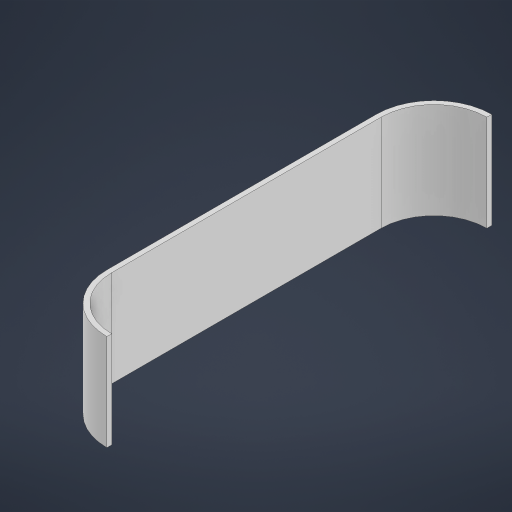
# Autodesk Inventor part: Pala
Saved by Autodesk Inventor 2023 (Build 270158000, 158)
## iProperties
Created: 2022-08-24
Part Number: Pala
Material: Generic
Document SubType Name: Modeling
Designer: river
Density: 1 g/cm^3
Appearance: Default
Author: river
Autodesk Inventor part; units mm, degrees
ref_plane "YZ Plane" through (0, 0, 0) normal (1, 0, 0) x (0, 1, 0)
ref_plane "XZ Plane" through (0, 0, 0) normal (0, 1, 0) x (-1, 0, 0)
ref_plane "XY Plane" through (0, 0, 0) normal (0, 0, 1) x (1, 0, 0)
sketch "Sketch1" plane through (0, 0, 0) normal (0, 1, 0) x (-1, 0, 0)
  line L0 (0, 0) -> (-30, 0)
  line L1 (-30, 0) -> (-30, -100)
  line L2 (-30, -100) -> (0, -100)
  line L3 (0, -100) -> (0, 0)
  line L4 (0, 0) -> (15, 0)
  line L5 (15, 0) -> (15, -55)
  line L6 (15, -55) -> (0, -55)
  line L7 (0, -55) -> (0, 0)
  circle A0 centre (7.5, 0) radius 2.5
  circle A1 centre (7.5, -20) radius 2.5
  circle A2 centre (7.5, -40) radius 2.5
  line L8 (0, -100) -> (0, -70)
  line L9 (0, -70) -> (-30, -70)
  circle A3 centre (-30, -70) radius 30
  circle A4 centre (-30, -70) radius 27.5
  line L10 (-2.5, -70) -> (-2.5, 0)
  point P0 (10, 0)
  point P1 (5, 0)
  point P2 (-30, -97.5)
  dimension "d12" = 55
  dimension "d2" = 30
  dimension "d3" = 100
  dimension "d4" = 15
  dimension "d5" = 55
  dimension "d6" = 5
  dimension "d7" = 5
  dimension "d8" = 20
  dimension "d9" = 5
  dimension "d10" = 40
  dimension "d11" = 30
  constraints: 22 end point, 4 parallel, 4 perpendicular, 4 point on line, 3 centre point, 2 coincident, 2 horizontal, 1 midpoint, 1 vertical, 6 other
  measures "d2" distance of L2.end L1.end
  measures "d3" distance of L1.end L0.end
  measures "d4" distance of L5.end L6.end
  measures "d5" distance of L4.end L5.end
  measures "d6" diameter of A0
  measures "d7" diameter of A1
  measures "d8" distance of A1.centre A0.centre
  measures "d9" diameter of A2
  measures "d10" distance from line of L4 A2.centre
  measures "d11" distance of L2.end L8.end
extrude "Extrusion1" add sketch "Sketch1" along normal blind 50 contours L3 A3 L10 L0 | L4 A0 L5 L6 L3 | A3 L9 L10 | A3 L1 A4 L9
sketch "Sketch2" plane through (0, 50, 0) normal (0, 1, 0) x (1, 0, 0)
  line L0 (-15, 55) -> (-15, 0) projected
  line L1 (0, 0) -> (-15, 0)
  line L2 (-15, 0) -> (-15, 55)
  line L3 (-15, 55) -> (0, 55)
  line L4 (0, 55) -> (0, 0)
  constraints: 8 end point, 2 parallel, 1 horizontal, 1 perpendicular
extrude "Extrusion2" cut sketch "Sketch2" against normal blind 16.8
mirror "Mirror1" about plane through (-5, 0, 0) normal (0, 0, 1) of "Extrusion1"
mirror "Mirror2" about plane through (-5, 0, 0) normal (0, 0, -1) of "Extrusion2"
sketch "Sketch3" plane through (0, 0, 0) normal (0, -1, 0) x (1, 0, 0)
  line L0 (0, -55) -> (-15, -55) projected
  line L1 (0, 0) -> (-15, 0)
  line L2 (-15, 0) -> (-15, -55)
  line L3 (-15, -55) -> (0, -55)
  line L4 (0, -55) -> (0, 0)
  constraints: 8 end point, 2 parallel, 1 horizontal, 1 perpendicular
extrude "Extrusion3" cut sketch "Sketch3" against normal blind 23.2
mirror "Mirror3" about plane through (-15, 0, 0) normal (0, 0, -1) of "Extrusion3"
body "Solid1"
